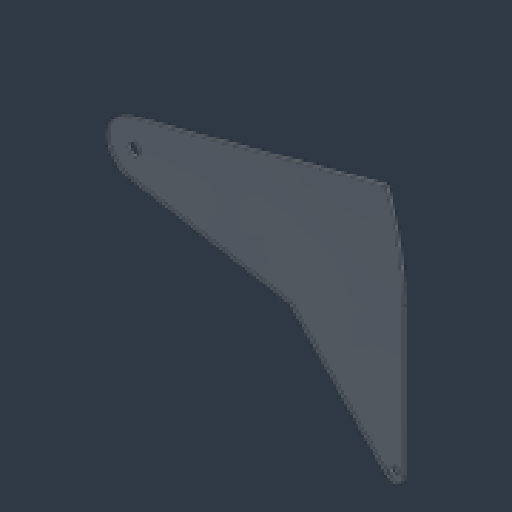
# Autodesk Inventor part: PLATE,ARM,DROPBAR
Saved by Autodesk Inventor 2026 (Build 300175050, 175E)
## iProperties
Created: 2026-04-04
Part Number: PLATE,ARM,DROPBAR
Material: Polycarbonate, Clear
Document SubType Name: Sheet Metal
Designer: Jthib
Mass: 120.082 g
Surface Area: 684.396 cm^2
Volume: 100.068 cm^3
Density: 1.2 g/cm^3
Sheet Metal Rule: Default
Appearance: Polycarbonate - Clear
Author: Jthib
Autodesk Inventor part; units mm, degrees
ref_plane "YZ Plane" through (0, 0, 0) normal (1, 0, 0) x (0, 1, 0)
ref_plane "XZ Plane" through (0, 0, 0) normal (0, 1, 0) x (-1, 0, 0)
ref_plane "XY Plane" through (0, 0, 0) normal (0, 0, 1) x (1, 0, 0)
sketch "Sketch1" plane through (0, 0, 0) normal (0, 0, 1) x (1, 0, 0)
  arc A0 (-6.574, 24.5345) -> (-4.4107, -25.0141) centre (0, 0) ccw
  line L0 (-4.4107, -25.0141) -> (146.1169, -51.5562)
  line L1 (146.1169, -51.5562) -> (237.6232, -146.3165)
  arc A1 (237.6232, -146.3165) -> (254, -139.7) centre (244.475, -139.7) ccw
  line L2 (-83.3652, 0) -> (314.9884, 0) construction
  line L3 (254, -139.7) -> (254, 0)
  arc A2 (254, 0) -> (237.5413, 89.945) centre (0, 0) ccw
  line L4 (237.5413, 89.945) -> (-6.574, 24.5345)
  dimension "d1" = 9.525
  dimension "d2" = 25.4
  dimension "d3" = 10
  dimension "d4" = 46.001
  dimension "d6" = 254
  dimension "d7" = 139.7
  dimension "d8" = 15
  measures "d1" radius of A1
  measures "d2" radius of A0
  measures "d3" angle of L2 L0
  measures "d4" angle of L2 L1
  measures "d6" distance from line of L3 point (0, 0)
  measures "d7" distance from line of L2 A1.centre
  measures "d8" angle of L2 L4
extrude "Plate1" add sketch "Sketch1" along normal blind 3.048
sketch "Sketch2" plane through (0, 0, 3.048) normal (0, 0, 1) x (1, 0, 0)
  point P0 (0, 0)
  point P1 (0, 0)
  constraints: 1 coincident
hole "Hole1" at (0, 0, 3.048) direction (0, 0, -1) diameter 9.525 end through all
sketch "Sketch3" plane through (0, 0, 3.048) normal (0, 0, 1) x (1, 0, 0)
  arc A0 (237.6232, -146.3165) -> (254, -139.7) centre (244.475, -139.7) ccw construction
  point P0 (0, 0)
  constraints: 1 coincident
hole "Hole2" at (244.475, -139.7, 3.048) direction (0, 0, -1) diameter 6.7564 end through all clearance for "Flat Head Machine Screw (82)" size "1/4" standard "Ansi Unified Screw Threads"
equation "\"d14\" = Thickness"
equation "\"d0\" = Thickness"
equation "\"BendRadius\" = Thickness"
equation "\"BendReliefWidth\" = Thickness"
equation "\"BendReliefDepth\" = 0.5 * Thickness"
equation "\"CornerReliefSize\" = 4 * Thickness"
equation "\"MinimumRemnant\" = 2 * Thickness"
equation "\"TransitionRadius\" = BendRadius"
equation "\"JacobiRadiusSize\" = BendRadius"
equation "\"GapSize\" = Thickness"
equation "\"Thickness\" = 3.048"
body "Solid1"
